Autodesk Fusion 360 part; units mm, degrees
(part 2 of 2)
equation "d614 = 3 mm - magnetDepth"
equation "d616 = buttonOD"
equation "d617 = ( 34.2 / 2 ) * 1 mm"
equation "d620 = ( 39.2 / 2 ) * 1 mm"
equation "d621 = buttonH"
equation "d624 = 39.2 mm - 0.5 mm"
equation "d625 = 34.2 mm - 0.5 mm"
equation "d850 = buttonBaseW"
equation "d853 = magnetDepth"
equation "d860 = 3 mm + magnetDepth"
equation "d862 = ( 38 / 2 ) * 1 mm"
equation "d863 = ( 33.5 / 2 ) * 1 mm"
equation "d864 = buttonOD"
equation "d867 = buttonH"
equation "buttonOD = 28 mm"
equation "buttonH = 15 mm"
equation "magnetDepth = -1.8 mm" comment "1.43 mm"
equation "buttonBaseW = 33.5 mm"

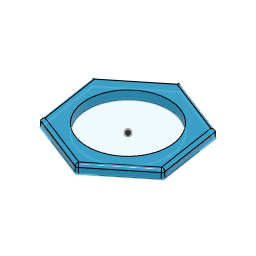
design "Button Aesthetic Ring"
Autodesk Fusion 360 part; units mm, degrees
sketch "Sketch1" plane through (0, 0, 0) normal (0, 1, 0) x (1, 0, 0)
  circle A0 centre (116.6706, -10) radius 14.5
  line L0 (137.33, -17.9988) -> (133.9274, 3.8922)
  line L1 (133.9274, 3.8922) -> (113.268, 11.8909)
  line L2 (113.268, 11.8909) -> (96.0112, -2.0012)
  line L3 (96.0112, -2.0012) -> (99.4138, -23.8922)
  line L4 (99.4138, -23.8922) -> (120.0732, -31.8909)
  line L5 (120.0732, -31.8909) -> (137.33, -17.9988)
  point P0 (116.6706, -10)
  dimension "d140" = 29
  measures "d140" diameter of A0
extrude "Extrude1" add sketch "Sketch1" along normal blind 3
fillet "Fillet1" radius 1 1 edges at (128.7016, 3, 24.9448)
fillet "Fillet2" radius 1 9 edges at (109.2051, 3, 27.6831) (119.7578, 2.7071, 31.7688) (120.0732, 1, 31.8909) (137.33, 1, 17.9988) (137.2781, 2.7071, 17.6646) (135.54, 3, 6.4828) (123.5977, 3, -7.8916) (97.7125, 3, 12.9467) (104.6396, 3, -4.9448)
equation "d140 = buttonOD + 1 mm"
equation "buttonOD = 28 mm"
